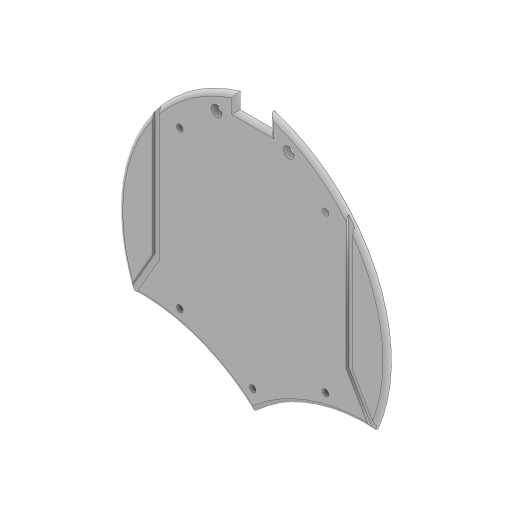
# Autodesk Inventor part: manta ray baseplate
Saved by Autodesk Inventor 2024 (Build 280153000, 153)
## iProperties
Created: 2024-01-10
Part Number: manta ray baseplate
Material: Generic
Document SubType Name: Modeling
Designer: chris
Density: 1 g/cm^3
Appearance: Default
Author: chris
Autodesk Inventor part; units mm, degrees
ref_plane "YZ Plane" through (0, 0, 0) normal (1, 0, 0) x (0, 1, 0)
ref_plane "XZ Plane" through (0, 0, 0) normal (0, 1, 0) x (-1, 0, 0)
ref_plane "XY Plane" through (0, 0, 0) normal (0, 0, 1) x (1, 0, 0)
sketch "Sketch2" plane through (0, 0, 0) normal (0, 0, 1) x (1, 0, 0)
  line L0 (-7.8424, 77.5) -> (-7.8424, 85)
  line L1 (0, 0) -> (0, -35)
  line L2 (0, -35) -> (0, -40)
  arc A0 (-7.8424, 85) -> (-56.4438, -19.47) centre (14.5186, 11.0571) ccw
  line L3 (-7.8424, 77.5) -> (0, 77.5)
  arc A1 (0, -40) -> (-56.4438, -19.47) centre (-52.7866, -97.2714) ccw
  line L4 (7.8424, 77.5) -> (7.8424, 85)
  arc A2 (56.4438, -19.47) -> (7.8424, 85) centre (-14.5186, 11.0571) ccw
  line L5 (7.8424, 77.5) -> (0, 77.5)
  arc A3 (56.4438, -19.47) -> (0, -40) centre (52.7866, -97.2714) ccw
  point P0 (-47.5, -35)
  point P1 (47.5, -35)
  dimension "d5" = 47.5
  dimension "d7" = 5
  dimension "d9" = 35
  dimension "d11" = 77.25
  constraints: 12 end point, 8 point on circle, 6 symmetric about line, 4 centre point, 3 vertical, 1 horizontal, 2 other
  measures "d5" distance of L1.end point (-47.5, -35)
  measures "d7" distance of L1.end L2.end
  measures "d9" distance of L1.start L1.end
  measures "d11" radius of A0
extrude "Extrusion1" add sketch "Sketch2" along normal blind 3
sketch "Sketch3" plane through (0, 0, 3) normal (0, 0, 1) x (1, 0, 0)
  arc A0 (56.4438, -19.47) -> (0, -40) centre (52.7866, -97.2714) ccw projected
  line L0 (0, -40) -> (0, -15)
  line L1 (0, -15) -> (-34, -15)
  line L2 (-34, -15) -> (-34, 58)
  line L3 (-34, 58) -> (34, 58)
  line L4 (34, 58) -> (34, -15)
  line L5 (34, -15) -> (0, -15)
  circle A1 centre (-34, 58) radius 1.5
  circle A2 centre (34, 58) radius 1.5
  circle A3 centre (-34, -15) radius 1.5
  circle A4 centre (34, -15) radius 1.5
  point P0 (0, 0)
  dimension "d20" = 25
  dimension "d21" = 34
  dimension "d22" = 73
  dimension "d23" = 68
  dimension "d24" = 3
  dimension "d25" = 3
  dimension "d26" = 3
  constraints: 12 end point, 5 perpendicular, 4 centre point, 4 coincident, 1 point on line, 1 vertical
  measures "d20" distance of L0.start L0.end
  measures "d21" distance of L0.end L1.end
  measures "d22" distance of L1.end L2.end
  measures "d23" distance of L2.end L3.end
  measures "d24" diameter of A1
  measures "d25" diameter of A2
  measures "d26" diameter of A3
extrude "Extrusion2" cut sketch "Sketch3" against normal through all contours A3 L2 L1 | L1 L2 A3 | A4 L4 L5 | L5 L4 A4 | A1 L3 L2 | L2 L3 A1 | A2 L3 L4 | L4 L3 A2
fillet "Fillet1" radius 2 14 edges at (-55.5229, 43.6417, 3) (-7.8424, 81.25, 3) (0, 77.5, 3) (7.8424, 81.25, 3) (55.5229, 43.6417, 3) (-26.1634, -24.0755, 3) (26.1634, -24.0755, 3) (26.1634, -24.0755, 0) (-26.1634, -24.0755, 0) (-55.5229, 43.6417, 0) (55.5229, 43.6417, 0) (-7.8424, 81.25, 0) (0, 77.5, 0) (7.8424, 81.25, 0)
sketch "Sketch4" plane through (0, 0, 3) normal (0, 0, 1) x (1, 0, 0)
  circle A0 centre (0, -30.3084) radius 1.5
  point P0 (0, -37.3084)
  dimension "d33" = 3
  constraints: 1 centre point
  measures "d33" diameter of A0
extrude "Extrusion3" cut sketch "Sketch4" against normal blind 10
sketch "Sketch5" plane through (0, 0, 3) normal (0, 0, 1) x (1, 0, 0)
  line L0 (-11.8424, 73.5) -> (-16.8424, 73.5)
  circle A0 centre (-16.8424, 73.5) radius 2.5
  arc A1 (-9.8424, 82.2548) -> (-51.9195, 46.3918) centre (14.5186, 11.0571) ccw
  line L1 (9.8424, 75.5) -> (-9.8424, 75.5)
  line L2 (0, 75.5) -> (0, 92.1707)
  circle A2 centre (16.8424, 73.5) radius 2.5
  arc A3 (51.9195, 46.3918) -> (9.8424, 82.2548) centre (-14.5186, 11.0571) ccw
  line L3 (-9.8424, 75.5) -> (9.8424, 75.5) projected
  line L4 (0, 75.5) -> (7.9828, 69.7684)
  point P0 (0, 0)
  dimension "d36" = 5
  dimension "d37" = 5
  constraints: 8 end point, 4 centre point, 4 point on circle, 2 midpoint, 1 coincident, 1 horizontal, 1 symmetric about line, 1 vertical, 1 other
  measures "d36" distance of L0.start L0.end
  measures "d37" diameter of A0
extrude "Extrusion4" cut sketch "Sketch5" against normal blind 10
sketch "Sketch6" plane through (0, 0, 3) normal (0, 0, 1) x (1, 0, 0)
  arc A0 (-7.8424, 85) -> (-56.4438, -19.47) centre (14.5186, 11.0571) ccw projected
  line L0 (-56.4438, -19.47) -> (-45.2028, 0)
  line L1 (-56.4438, -19.47) -> (-19.8564, -19.47) construction
  line L2 (-45.2028, 0) -> (-45.2028, 60.0563)
  line L3 (-46.7028, 58.1687) -> (-46.7028, 0.4019)
  line L4 (-46.7028, 0.4019) -> (-57.1689, -17.7259)
  line L5 (-43.7028, -0.4019) -> (-53.8457, -17.97)
  line L6 (-43.7028, -0.4019) -> (-54.7117, -19.47)
  arc A1 (0, -40) -> (-56.4438, -19.47) centre (-52.7866, -97.2714) ccw projected
  line L7 (-43.7028, -0.4019) -> (-43.7028, 61.8295)
  line L8 (-9.8424, 75.5) -> (9.8424, 75.5) projected
  line L9 (0, 75.5) -> (0, 95.6739)
  arc A2 (56.4438, -19.47) -> (7.8424, 85) centre (-14.5186, 11.0571) ccw
  line L10 (56.4438, -19.47) -> (45.2028, 0)
  line L11 (56.4438, -19.47) -> (19.8564, -19.47) construction
  line L12 (45.2028, 0) -> (45.2028, 60.0563)
  line L13 (46.7028, 58.1687) -> (46.7028, 0.4019)
  line L14 (46.7028, 0.4019) -> (57.1689, -17.7259)
  line L15 (43.7028, -0.4019) -> (53.8457, -17.97)
  line L16 (43.7028, -0.4019) -> (54.7117, -19.47)
  arc A3 (56.4438, -19.47) -> (0, -40) centre (52.7866, -97.2714) ccw
  line L17 (43.7028, -0.4019) -> (43.7028, 61.8295)
  point P0 (0, 0)
  point P1 (54.6754, -19.407)
  point P2 (-54.6754, -19.407)
  dimension "d41" = 60
  dimension "d42" = 1.5
  constraints: 34 end point, 14 symmetric about line, 12 point on circle, 3 vertical, 2 centre point, 2 point on line, 1 horizontal, 1 midpoint, 2 other
  measures "d41" angle of L1 L0
  measures "d42" distance between parallel lines of L0 L4
extrude "Extrusion5" cut sketch "Sketch6" against normal blind 1 contours L7 L5 L6 A1 L0 L2 A0 | L2 L0 A0 L4 L3 | L10 L12 A2 L13 L14 | A3 L16 L15 L17 A2 L12 L10
body "Solid1"
